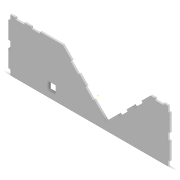
# Autodesk Inventor part: Fondo
Saved by Autodesk Inventor 2022 (Build 260153000, 153)
## iProperties
Created: 2022-06-06
Part Number: Fondo
Material: Generic
Document SubType Name: Modeling
Designer: ADMIN
Density: 1 g/cm^3
Appearance: Default
Author: ADMIN
Autodesk Inventor part; units mm, degrees
ref_plane "YZ Plane" through (0, 0, 0) normal (1, 0, 0) x (0, 1, 0)
ref_plane "XZ Plane" through (0, 0, 0) normal (0, 1, 0) x (-1, 0, 0)
ref_plane "XY Plane" through (0, 0, 0) normal (0, 0, 1) x (1, 0, 0)
sketch "Sketch1" plane through (0, 0, 0) normal (0, 0, 1) x (1, 0, 0)
  line L0 (200, -75) -> (-250, -75) projected
  line L1 (200, 75) -> (200, -75) projected
  line L2 (-250, 75) -> (-235, 75) projected
  line L3 (-250, -75) -> (-250, 75) projected
  line L4 (-255, -10) -> (-255, -60) projected
  line L5 (-255, -60) -> (-250, -60) projected
  line L6 (-250, -10) -> (-250, -60) projected
  line L7 (-255, -10) -> (-250, -10) projected
  line L8 (-255, 60) -> (-255, 10) projected
  line L9 (-255, 10) -> (-250, 10) projected
  line L10 (-250, 60) -> (-250, 10) projected
  line L11 (-255, 60) -> (-250, 60) projected
  line L12 (200, 60) -> (200, 10) projected
  line L13 (200, 10) -> (205, 10) projected
  line L14 (205, 60) -> (205, 10) projected
  line L15 (200, 60) -> (205, 60) projected
  line L16 (200, -10) -> (200, -60) projected
  line L17 (200, -60) -> (205, -60) projected
  line L18 (205, -10) -> (205, -60) projected
  line L19 (200, -10) -> (205, -10) projected
  line L20 (150, 75) -> (162.5, 75) projected
  line L21 (25, -50) -> (60.3553, -14.6447) projected
  line L22 (-100, 75) -> (-73.9949, 48.9949) projected
  line L23 (-10.3553, -14.6447) -> (-13.8909, -18.1802) projected
  line L24 (-13.8909, -18.1802) -> (-35.1041, 3.033) projected
  line L25 (-35.1041, 3.033) -> (-31.5685, 6.5685) projected
  line L26 (-52.7817, 27.7817) -> (-31.5685, 6.5685) projected
  line L27 (-52.7817, 27.7817) -> (-56.3173, 24.2462) projected
  line L28 (-56.3173, 24.2462) -> (-77.5305, 45.4594) projected
  line L29 (-77.5305, 45.4594) -> (-73.9949, 48.9949) projected
  line L30 (123.9949, 48.9949) -> (150, 75) projected
  line L31 (123.9949, 48.9949) -> (127.5305, 45.4594) projected
  line L32 (127.5305, 45.4594) -> (106.3173, 24.2462) projected
  line L33 (106.3173, 24.2462) -> (102.7817, 27.7817) projected
  line L34 (81.5685, 6.5685) -> (102.7817, 27.7817) projected
  line L35 (81.5685, 6.5685) -> (85.1041, 3.033) projected
  line L36 (85.1041, 3.033) -> (63.8909, -18.1802) projected
  line L37 (63.8909, -18.1802) -> (60.3553, -14.6447) projected
  line L38 (-10.3553, -14.6447) -> (25, -50) projected
  line L39 (-210, 75) -> (-210, 70) projected
  line L40 (-210, 70) -> (-235, 70) projected
  line L41 (-235, 70) -> (-235, 75) projected
  line L42 (187.5, 75) -> (200, 75) projected
  line L43 (187.5, 75) -> (187.5, 70) projected
  line L44 (187.5, 70) -> (162.5, 70) projected
  line L45 (162.5, 70) -> (162.5, 75) projected
  line L46 (-165, 75) -> (-100, 75) projected
  line L47 (-165, 75) -> (-165, 70) projected
  line L48 (-165, 70) -> (-190, 70) projected
  line L49 (-190, 70) -> (-190, 75) projected
  line L50 (-210, 75) -> (-190, 75) projected
  point P0 (0, 0)
extrude "Extrusion1" add sketch "Sketch1" along normal blind 5
sketch "Sketch2" plane through (0, 0, 5) normal (0, 0, 1) x (1, 0, 0)
  point P0 (0, 0)
sketch "Sketch4" plane through (0, 0, 5) normal (0, 0, 1) x (1, 0, 0)
  line L0 (200, -60) -> (205, -60) projected
  line L1 (205, -60) -> (205, -10) projected
  line L2 (205, -10) -> (200, -10) projected
  line L3 (200, -10) -> (200, 10) projected
  line L4 (200, 10) -> (205, 10) projected
  line L5 (205, 10) -> (205, 60) projected
  line L6 (205, 60) -> (200, 60) projected
  line L7 (200, 60) -> (200, 75) projected
  line L8 (200, 75) -> (187.5, 75) projected
  line L9 (187.5, 75) -> (187.5, 70) projected
  line L10 (187.5, 70) -> (162.5, 70) projected
  line L11 (162.5, 70) -> (162.5, 75) projected
  line L12 (162.5, 75) -> (150, 75) projected
  line L13 (150, 75) -> (123.9949, 48.9949) projected
  line L14 (123.9949, 48.9949) -> (127.5305, 45.4594) projected
  line L15 (127.5305, 45.4594) -> (106.3173, 24.2462) projected
  line L16 (106.3173, 24.2462) -> (102.7817, 27.7817) projected
  line L17 (102.7817, 27.7817) -> (81.5685, 6.5685) projected
  line L18 (81.5685, 6.5685) -> (85.1041, 3.033) projected
  line L19 (85.1041, 3.033) -> (63.8909, -18.1802) projected
  line L20 (63.8909, -18.1802) -> (60.3553, -14.6447) projected
  line L21 (60.3553, -14.6447) -> (25, -50) projected
  line L22 (25, -50) -> (-10.3553, -14.6447) projected
  line L23 (-10.3553, -14.6447) -> (-13.8909, -18.1802) projected
  line L24 (-13.8909, -18.1802) -> (-35.1041, 3.033) projected
  line L25 (-35.1041, 3.033) -> (-31.5685, 6.5685) projected
  line L26 (-31.5685, 6.5685) -> (-52.7817, 27.7817) projected
  line L27 (-52.7817, 27.7817) -> (-56.3173, 24.2462) projected
  line L28 (-56.3173, 24.2462) -> (-77.5305, 45.4594) projected
  line L29 (-77.5305, 45.4594) -> (-73.9949, 48.9949) projected
  line L30 (-73.9949, 48.9949) -> (-100, 75) projected
  line L31 (-100, 75) -> (-165, 75) projected
  line L32 (-165, 75) -> (-165, 70) projected
  line L33 (-165, 70) -> (-190, 70) projected
  line L34 (-190, 70) -> (-190, 75) projected
  line L35 (-190, 75) -> (-210, 75) projected
  line L36 (-210, 75) -> (-210, 70) projected
  line L37 (-210, 70) -> (-235, 70) projected
  line L38 (-235, 70) -> (-235, 75) projected
  line L39 (-235, 75) -> (-250, 75) projected
  line L40 (-250, 75) -> (-250, 60) projected
  line L41 (-250, 60) -> (-255, 60) projected
  line L42 (-255, 60) -> (-255, 10) projected
  line L43 (-255, 10) -> (-250, 10) projected
  line L44 (-250, 10) -> (-250, -10) projected
  line L45 (-250, -10) -> (-255, -10) projected
  line L46 (-255, -10) -> (-255, -60) projected
  line L47 (-255, -60) -> (-250, -60) projected
  line L48 (-250, -60) -> (-250, -75) projected
  line L49 (-250, -75) -> (200, -75) projected
  line L50 (200, -75) -> (200, -60) projected
  line L51 (-140, -35) -> (-120, -35)
  line L52 (-120, -35) -> (-120, -55)
  line L53 (-120, -55) -> (-140, -55)
  line L54 (-140, -55) -> (-140, -35)
  point P0 (0, 0)
  dimension "d4" = 20
  dimension "d5" = 20
  dimension "d6" = 20
  dimension "d7" = 110
  constraints: 8 end point, 2 parallel, 1 horizontal, 1 perpendicular
  measures "d4" distance of L52.end L53.end
  measures "d5" distance of L51.end L52.end
  measures "d6" distance between parallel lines of L49 L53
  measures "d7" distance between parallel lines of L48 L54
extrude "Extrusion3" cut sketch "Sketch4" against normal blind 10 contours L51 L52 L53 L54
body "Solid1"
